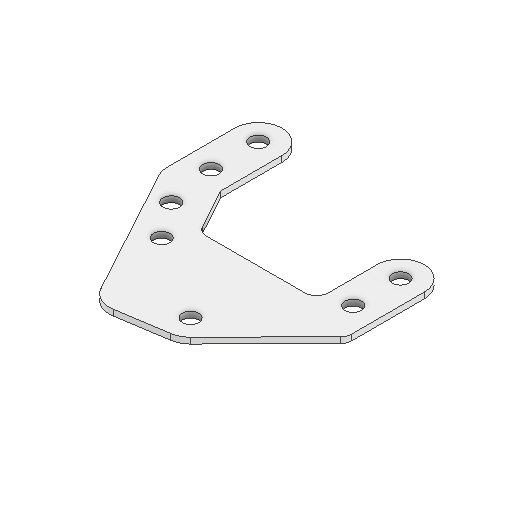
# Autodesk Inventor part: Ring Funnel
Saved by Autodesk Inventor 2025 (Build 290162000, 162)
## iProperties
Created: 2024-12-17
Part Number: Ring Funnel
Material: Acetal Resin, White
Document SubType Name: Modeling
Designer: Averey Ku
Density: 1.425 g/cm^3
Appearance: Smooth - White
Mass: 3.11762 g
Surface Area: 32.8414 cm^2
Volume: 2.1878 cm^3
d0: 0.172 in
d2: 0.500 in
d3: 0.250 in
d4: 0.500 in
d5: 0.172 in
d6: 0.172 in
d9: 0.250 in
d10: 1.250 in
d11: 1.469 in
d16: 0.250 in
d18: 0.125 in
d21: 0.188 in
d22: 0.125 in
d23: 0.500 in
d24: 0.500 in
d25: 0.250 in
d26: 0.525 in
Author: Averey Ku
Autodesk Inventor part; units mm, degrees
ref_plane "YZ Plane" through (0, 0, 0) normal (1, 0, 0) x (0, 1, 0)
ref_plane "XZ Plane" through (0, 0, 0) normal (0, 1, 0) x (-1, 0, 0)
ref_plane "XY Plane" through (0, 0, 0) normal (0, 0, 1) x (1, 0, 0)
sketch "main" plane through (0, 0, 0) normal (0, 0, 1) x (1, 0, 0)
  circle A0 centre (12.325875, 33.112504) radius 2.1844
  line L0 (25.390984, 29.120631) -> (25.316771, 29.135118)
  line L1 (20.04973, 41.835118) -> (13.667964, 35.453352) construction
  arc A1 (20.04973, 41.835118) -> (17.011045, 41.065244) centre (20.04973, 35.453352) ccw
  circle A2 centre (25.38373, 35.485118) radius 2.1844
  line L2 (20.04973, 41.835118) -> (29.074911, 41.835118) construction
  arc A3 (25.38373, 41.835118) -> (25.38373, 41.835118) centre (25.38373, 35.485118) ccw
  circle A4 centre (12.68373, -15.314882) radius 2.1844
  circle A5 centre (-11.92252, 3.735118) radius 2.1844
  arc A6 (-18.198047, 2.765449) -> (-16.395825, -0.77177) centre (-11.92252, 3.735118) ccw
  line L3 (-20.257316, 16.092677) -> (-18.198047, 2.765449)
  line L4 (12.391865, -8.964882) -> (25.38373, -8.964882)
  circle A7 centre (25.38373, -15.314882) radius 2.1844
  arc A8 (25.38373, -21.664882) -> (25.38373, -8.964882) centre (25.38373, -15.314882) ccw
  line L5 (5.962319, -21.664882) -> (25.38373, -21.664882)
  line L6 (3.725666, -20.743326) -> (-16.395825, -0.77177)
  line L7 (21.760398, 29.194623) -> (10.880086, 23.303233)
  line L8 (-17.005348, 22.646303) -> (17.011045, 41.065244)
  circle A9 centre (2.776273, 26.136374) radius 2.1844
  arc A10 (-17.005348, 22.646303) -> (-20.257316, 16.092677) centre (-13.981788, 17.062345) ccw
  line L9 (9.216865, -5.789882) -> (9.216865, 20.511254)
  arc A11 (9.216865, -5.789882) -> (12.391865, -8.964882) centre (12.391865, -5.789882) ccw
  arc A12 (10.880086, 23.303233) -> (9.216865, 20.511254) centre (12.391865, 20.511254) ccw
  arc A13 (3.725666, -20.743326) -> (5.962319, -21.664882) centre (5.962319, -18.489882) ccw
  arc A14 (38.08373, 29.135118) -> (38.08373, 41.835118) centre (38.08373, 35.485118) ccw
  line L10 (20.04973, 41.835118) -> (38.08373, 41.835118)
  line L11 (21.650503, 29.135118) -> (38.08373, 29.135118)
  circle A15 centre (38.08373, 35.485118) radius 2.184401
  point P0 (7.427211, 10.378199)
  point P1 (19.03373, 40.819118)
  point P2 (-20.9407, 20.515419)
  point P3 (9.216865, -8.964882)
  point P4 (-30.17877, -11.346132)
  dimension "d0" = 4.3688
  dimension "d2" = 12.7
  dimension "d3" = 6.35
  dimension "d4" = 12.7
  dimension "d5" = 4.3688
  dimension "d6" = 4.3688
  dimension "d9" = 6.35
  dimension "d10" = 31.75
  dimension "d11" = 37.30625
  dimension "d16" = 6.35
  dimension "d18" = 3.175
  dimension "d21" = 4.7625
  dimension "d22" = 3.175
  dimension "d23" = 12.7
  dimension "d24" = 12.7
  dimension "d25" = 6.35
  dimension "d26" = 13.32723
  measures "d0" diameter of A5
  measures "d2" diameter of A8
  measures "d3" radius of A10
  measures "d4" distance between parallel lines of L8 L7
  measures "d5" diameter of A9
  measures "d6" diameter of A0
  measures "d9" radius of A6
  measures "d10" vertical distance of A5.centre A2.centre
  measures "d11" horizontal distance of A5.centre A2.centre
  measures "d16" distance from line of L8 A9.centre
  measures "d18" radius of A11
  measures "d21" distance from line of L8 A0.centre
  measures "d22" radius of A13
  measures "d23" diameter of A14
  measures "d24" distance of A2.centre A15.centre
  measures "d25" radius of A14
  measures "d26" vertical distance of A5.centre A10.centre
sketch "Sketch1" plane through (0, 0, 0) normal (0, 1, 0) x (-1, 0, 0)
  circle A0 centre (-2.387595, 13.055125) radius 2.1844
  line L0 (-6.364475, -0.014556) -> (-6.350073, 0.059673)
  line L1 (6.343876, 5.341282) -> (-0.045209, 11.715722) construction
  arc A1 (6.343876, 5.341282) -> (5.570516, 8.379082) centre (-0.037886, 5.33396) ccw
  circle A2 centre (0, 0) radius 2.1844
  line L2 (6.343876, 5.341282) -> (6.354231, -3.683892) construction
  arc A3 (6.349996, 0.007286) -> (6.349996, 0.007286) centre (0, 0) ccw
  circle A4 centre (-50.814538, 12.641705) radius 2.1844
  circle A5 centre (-31.792784, 37.269796) radius 2.1844
  arc A6 (-32.769652, 43.544207) -> (-36.304801, 41.737927) centre (-31.792784, 37.269796) ccw
  line L3 (-19.444796, 45.618765) -> (-32.769652, 43.544207)
  line L4 (-44.464877, 12.940855) -> (-44.449971, -0.051001)
  circle A7 centre (-50.799967, -0.058287) radius 2.1844
  arc A8 (-57.149962, -0.065573) -> (-44.449971, -0.051001) centre (-50.799967, -0.058287) ccw
  line L5 (-57.172246, 19.355826) -> (-57.149962, -0.065573)
  line L6 (-56.253257, 21.593534) -> (-36.304801, 41.737927)
  line L7 (-6.294648, 3.616113) -> (-12.198518, 14.489658)
  line L8 (-12.887443, 42.374319) -> (5.570516, 8.379082)
  circle A9 centre (-9.374677, 22.596715) radius 2.1844
  arc A10 (-12.887443, 42.374319) -> (-19.444796, 45.618765) centre (-18.467928, 39.344355) ccw
  line L9 (-41.293522, 16.119496) -> (-14.992403, 16.149674)
  arc A11 (-41.293522, 16.119496) -> (-44.464877, 12.940855) centre (-41.289879, 12.944498) ccw
  arc A12 (-12.198518, 14.489658) -> (-14.992403, 16.149674) centre (-14.98876, 12.974676) ccw
  arc A13 (-56.253257, 21.593534) -> (-57.172246, 19.355826) centre (-53.997248, 19.359469) ccw
  arc A14 (-6.335424, -12.707278) -> (6.364568, -12.692706) centre (0.014572, -12.699992) ccw
  line L10 (6.343876, 5.341282) -> (6.364568, -12.692706)
  line L11 (-6.354279, 3.725939) -> (-6.335424, -12.707278)
  circle A15 centre (0.014572, -12.699992) radius 2.184401
  point P0 (0, 0)
  constraints: 1 other
extrude "Extrusion1" add sketch "Sketch1" along normal blind 1.5875
body "Solid1"
